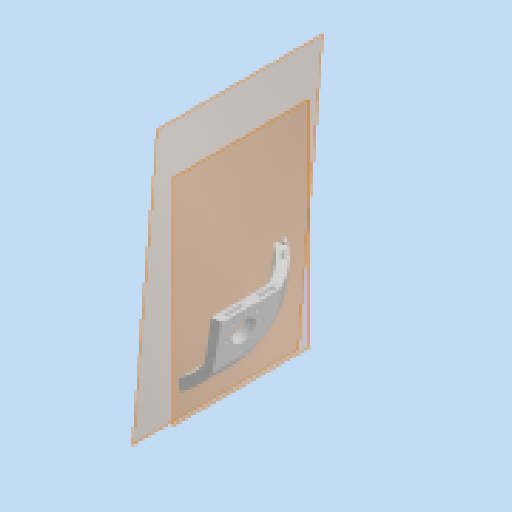
# Autodesk Inventor part: eggshellCorePrinted
Saved by Autodesk Inventor 2023 (Build 270158000, 158)
## iProperties
Created: 2026-03-19
Part Number: eggshellCorePrinted
Material: GFRC
Document SubType Name: Modeling
Designer: Nathann
Density: 1.7 g/cm^3
Appearance: Flat - Polished Gray
Mass: 25539 g
Surface Area: 11826.8 cm^2
Volume: 15023 cm^3
Author: Nathann
Autodesk Inventor part; units mm, degrees
ref_plane "XZ Plane" through (0, 0, 0) normal (0, 1, 0) x (-1, 0, 0)
ref_plane "XY Plane" through (0, 0, 0) normal (0, 0, 1) x (1, 0, 0)
sketch "Sketch1" plane through (0, 0, 0) normal (0, 0, 1) x (1, 0, 0)
  ellipse E0 centre (0, 0) end of major axis (0, 330) minor radius 450 (0, -330) -> (0, 330) ccw
  ellipse E1 centre (0, 0) end of major axis (420, 0) minor radius 300 (0, -300) -> (0, 300) ccw
  line L0 (0, 300) -> (0, 330)
  line L1 (0, -300) -> (0, -330)
  line L2 (420, 0) -> (450, 0)
  dimension "d0" = 420
  dimension "d1" = 450
  dimension "d2" = 300
  dimension "d3" = 330
  constraints: 6 end point, 2 coincident, 2 point on line, 1 horizontal, 10 other
extrude "Extrusion1" add sketch "Sketch1" along normal blind 80
sketch "Sketch2" plane through (0, 0, 80) normal (0, 0, 1) x (1, 0, 0)
  line L0 (0, 0) -> (451.5059, 0)
  ellipse E0 centre (0, 0) end of major axis (-450, 0) minor radius 330 (0, -330) -> (0, 330) ccw projected
  line L1 (0, 330) -> (0, 300) projected
  ellipse E1 centre (0, 0) end of major axis (-420, 0) minor radius 300 (0, -300) -> (0, 300) ccw projected
  line L2 (0, -300) -> (0, -330) projected
  point P0 (420, 0)
  point P1 (450, 0)
  constraints: 2 end point, 1 horizontal, 2 other
revolve "Revolution1" add sketch "Sketch2" angle 180 about axis through (0, 0, 80) along (1, 0, 0) contours E1 L1 E0 L0
sketch "Sketch3" plane through (0, 0, 0) normal (0, 0, -1) x (-1, 0, 0)
  ellipse E0 centre (0, 0) end of major axis (420, 0) minor radius 300 (0, 300) -> (0, -300) ccw projected
  line L0 (-410.6033, 63.104) -> (-375.8737, -133.8576)
  line L1 (-375.8737, -133.8576) -> (-428.5073, -143.1383)
  line L2 (-428.5073, -143.1383) -> (-456.291, 14.4309)
  line L3 (0, 300) -> (0, -300) projected
  ellipse E1 centre (0, 0) end of major axis (450, 0) minor radius 330 (0, 330) -> (0, -330) ccw projected
  line L4 (-456.291, 14.4309) -> (-439.6592, 70.3382)
  line L5 (-428.5073, -143.1383) -> (-336.4493, -219.1451)
  line L6 (-336.4493, -219.1451) -> (-375.8737, -133.8576)
  line L7 (-410.6033, 63.104) -> (-439.6592, 70.3382)
  line L8 (-393.2385, -35.3768) -> (260.9914, 90.2506)
  line L9 (260.9914, 90.2506) -> (260.9914, 44.7879)
  line L10 (260.9914, 44.7879) -> (0, 40.1342)
  dimension "d8" = 200
  dimension "d9" = 10
  dimension "d12" = 45.4627
  dimension "d13" = 160
  constraints: 20 end point, 2 perpendicular, 2 point on line, 1 midpoint, 1 vertical, 9 other
  measures "d8" distance of L0.start L0.end
  measures "d9" angle of L3 L0
  measures "d12" distance of L8.end L9.end
  measures "d13" distance of L1.end L2.end
extrude "Extrusion2" add sketch "Sketch3" against normal blind 190 contours L0 E0
ref_plane "Work Plane1" through (440.1475, 57.8945, 0) normal (-0.9848078, 0.1736482, 0) x (0, 0, 1)
sketch "Sketch5" plane through (440.1475, 57.8945, 0) normal (-0.9848078, 0.1736482, 0) x (0, 0, 1)
  line L0 (80, -458.4323) -> (80, -55.3041) projected
  circle A0 centre (80, -117.2866) radius 241.1725
  point P0 (0, -133.4458)
  constraints: 1 centre point, 1 point on line
extrude "Extrusion4" cut sketch "Sketch5" against normal blind 160
sketch "Sketch6" plane through (0, -330, 0) normal (-1, 0, 0) x (0, 0, 1)
  line L0 (0, 30) -> (0, 0) projected
  line L1 (0, 0) -> (80, 0) projected
  arc A0 (80, 0) -> (80, 660) centre (80, 330) ccw projected
  line L2 (0, 660) -> (80, 660) projected
  line L3 (0, 660) -> (0, 630) projected
  line L4 (0, 630) -> (80, 630) projected
  arc A1 (80, 30) -> (80, 630) centre (80, 330) ccw projected
  line L5 (0, 30) -> (80, 30) projected
  arc A2 (80, -50) -> (80, 710) centre (80, 330) ccw
  line L6 (80, -50) -> (-50, -50)
  line L7 (-50, -50) -> (-50, 80)
  line L8 (-50, 80) -> (80, 80)
  arc A3 (80, 80) -> (80, 580) centre (80, 330) ccw
  line L9 (80, 580) -> (-50, 580)
  line L10 (-50, 580) -> (-50, 710)
  line L11 (-50, 710) -> (80, 710)
  line L12 (0, 660) -> (0, 710)
  line L13 (0, 0) -> (0, -50)
  line L14 (80, 330) -> (410, 330)
  circle A4 centre (435, 330) radius 4.25
  circle A5 centre (426.0994, 408.9949) radius 4.25
  circle A6 centre (399.844, 484.0287) radius 4.25
  circle A7 centre (357.5502, 551.3389) radius 4.25
  circle A8 centre (301.3389, 607.5502) radius 4.25
  circle A9 centre (234.0288, 649.8439) radius 4.25
  circle A10 centre (158.995, 676.0994) radius 4.25
  circle A11 centre (80, 685) radius 4.25
  circle A12 centre (435, 330) radius 4.25
  circle A13 centre (426.0994, 251.0051) radius 4.25
  circle A14 centre (399.844, 175.9713) radius 4.25
  circle A15 centre (357.5502, 108.6611) radius 4.25
  circle A16 centre (301.3389, 52.4498) radius 4.25
  circle A17 centre (234.0288, 10.1561) radius 4.25
  circle A18 centre (158.995, -16.0994) radius 4.25
  circle A19 centre (80, -25) radius 4.25
  point P0 (0, 330)
  point P1 (460, 330)
  point P2 (80, -50)
  point P3 (460, 330)
  point P4 (439.25, 330)
  point P5 (430.75, 330)
  dimension "d19" = 50
  dimension "d22" = 8.5
  dimension "d25" = 90
  dimension "d27" = 25
  dimension "d28" = 0
  constraints: 18 centre point, 18 end point, 10 symmetric about line, 6 point on circle, 3 point on line, 1 perpendicular, 30 other
  measures "d19" distance between parallel lines of L1 L6
  measures "d22" diameter of A4
  measures "d27" distance of point (460, 330) A4.centre
  measures "d28" vertical distance of point (460, 330) A4.centre
extrude "Extrusion5" add sketch "Sketch6" against normal blind 10 contours L5 A1 L14 A0 L1 L0 | L1 A0 L2 L12 L11 A2 L6 L13 | A1 L4 L3 L2 A0 L14
ref_plane "Work Plane2" through (0, 0, 0) normal (0, 0, -1) x (-1, 0, 0)
mirror "Mirror1" about plane through (0, 0, 0) normal (0, 0, -1) of "Extrusion5", "Extrusion4", "Extrusion2", "Revolution1", "Extrusion1"
sketch "Sketch7" plane through (0, 0, 0) normal (0, 0, -1) x (-1, 0, 0)
  line L0 (-663.6694, -741.8919) -> (123.4449, -741.8919)
  line L1 (123.4449, -741.8919) -> (123.4449, 592.7802)
  line L2 (123.4449, 592.7802) -> (-663.6694, 592.7802)
  line L3 (-663.6694, 592.7802) -> (-663.6694, -741.8919)
  point P0 (0, 0)
  constraints: 8 end point, 2 parallel, 1 horizontal, 1 perpendicular
extrude "Extrusion6" cut sketch "Sketch7" against normal blind 1000
sketch "Sketch8" plane through (440.1475, 57.8945, 0) normal (0.9848078, -0.1736482, 0) x (0, 0, -1)
  line L0 (0, 6.7266) -> (80, 6.7266) projected
  line L1 (80, -205.7359) -> (0, -205.7359) projected
  circle A0 centre (80, -125.7359) radius 35
  line L2 (0, 6.7266) -> (0, -205.7359) projected
  circle A1 centre (80, -180.7359) radius 4.5
  circle A2 centre (118.8909, -164.6268) radius 4.5
  circle A3 centre (135, -125.7359) radius 4.5
  circle A4 centre (118.8909, -86.845) radius 4.5
  circle A5 centre (80, -70.7359) radius 4.5
  circle A6 centre (41.1091, -86.845) radius 4.5
  circle A7 centre (25, -125.7359) radius 4.5
  circle A8 centre (41.1091, -164.6268) radius 4.5
  point P0 (80.0002, -99.5046)
  dimension "d42" = 80
  dimension "d43" = 70
  dimension "d44" = 80
  dimension "d45" = 9
  dimension "d46" = 55
  dimension "d49" = 360
  constraints: 9 centre point, 1 vertical alignment, 17 other
  measures "d42" distance from line of L2 A0.centre
  measures "d43" diameter of A0
  measures "d44" distance from line of L1 A0.centre
  measures "d45" diameter of A1
  measures "d46" distance of A0.centre A1.centre
extrude "Extrusion7" cut sketch "Sketch8" against normal blind 50
ref_plane "Work Plane3" through (10, -2381.5933, 0) normal (0.9961947, -0.0871557, 0) x (0, 0, 1)
ref_plane "Work Plane4" through (300, 0, 0) normal (1, 0, 0) x (0, 1, 0)
sketch "Sketch10" plane through (300, 0, 0) normal (1, 0, 0) x (0, 1, 0)
  line L0 (-646.9693, -896.2791) -> (523.3446, -896.2791)
  line L1 (523.3446, -896.2791) -> (523.3446, 327.6055)
  line L2 (523.3446, 327.6055) -> (-646.9693, 327.6055)
  line L3 (-646.9693, 327.6055) -> (-646.9693, -896.2791)
  point P0 (0, 0)
  constraints: 8 end point, 2 parallel, 1 horizontal, 1 perpendicular
extrude "Extrusion9" cut sketch "Sketch10" against normal through all
sketch "Sketch11" plane through (300, 0, 0) normal (1, 0, 0) x (0, 1, 0)
  line L0 (384.5563, 0) -> (0.9675, 0)
  line L1 (0.9675, 0) -> (0.9675, -396.3946)
  line L2 (0.9675, -396.3946) -> (384.5563, -396.3946)
  line L3 (384.5563, -396.3946) -> (384.5563, 0)
  line L4 (245.9675, -80) -> (245.9675, 0) projected
  dimension "d58" = 245
  constraints: 8 end point, 2 parallel, 1 horizontal, 1 perpendicular
  measures "d58" distance between parallel lines of L1 L4
extrude "Extrusion10" cut sketch "Sketch11" along normal through all
sketch "Sketch12" plane through (399.647, 0.9675, 0) normal (0, 1, 0) x (1, 0, 0)
  line L0 (20.4628, 25) -> (10.4628, 25)
  line L1 (10.4628, 25) -> (10.4628, 75)
  line L2 (10.4628, 75) -> (20.4628, 75)
  line L3 (20.4628, 75) -> (20.4628, 25)
  line L4 (20.4628, 175) -> (10.4628, 175)
  line L5 (10.4628, 175) -> (10.4628, 125)
  line L6 (10.4628, 125) -> (20.4628, 125)
  line L7 (20.4628, 125) -> (20.4628, 175)
  line L8 (-61.515, 285.7558) -> (-26.1597, 250.4004)
  line L9 (-26.1597, 250.4004) -> (-33.2307, 243.3294)
  line L10 (-33.2307, 243.3294) -> (-68.5861, 278.6847)
  line L11 (-68.5861, 278.6847) -> (-61.515, 285.7558)
  line L12 (30.4628, 0) -> (0, 0) projected
  line L13 (30.4628, 177.0216) -> (30.4628, 0) projected
  line L14 (0, 0) -> (0, 172.2521) projected
  line L15 (-71.4051, 309.788) -> (19.6676, 218.7153)
  line L16 (-99.647, 0) -> (-23.7733, 0) projected
  line L17 (-36.7663, 275.1492) -> (-26.3833, 285.5322)
  point P0 (-399.647, 0)
  point P1 (0, 160)
  dimension "d59" = 10
  dimension "d60" = 10
  dimension "d61" = 50
  dimension "d62" = 50
  dimension "d63" = 10
  dimension "d64" = 50
  dimension "d65" = 25
  dimension "d66" = 50
  dimension "d67" = 10
  dimension "d68" = 10.4628
  dimension "d69" = 10
  dimension "d71" = 45
  dimension "d72" = 10
  dimension "d73" = 25
  constraints: 28 end point, 7 parallel, 4 perpendicular, 2 horizontal, 2 point on line, 3 other
  measures "d59" distance of L1.end L2.end
  measures "d60" distance of L4.start L4.end
  measures "d61" distance of L6.end L4.start
  measures "d62" distance of L2.end L0.start
  measures "d63" distance of L8.end L9.end
  measures "d64" distance of L8.start L8.end
  measures "d65" distance between parallel lines of L12 L0
  measures "d66" distance between parallel lines of L2 L6
  measures "d67" distance between parallel lines of L13 L3
  measures "d68" distance between parallel lines of L14 L1
  measures "d69" distance between parallel lines of L13 L7
  measures "d71" angle of L16 L15
  measures "d72" distance from line of L8 L17.start
  measures "d73" distance between parallel lines of L9 L17
extrude "Extrusion11" cut sketch "Sketch12" along normal blind 20 and the other way blind 20
sketch "Sketch13" plane through (300, 0, 0) normal (-1, 0, 0) x (0, 0, 1)
  line L0 (-25, -220.9675) -> (-75, -220.9675)
  line L1 (-75, -220.9675) -> (-75, -230.9675)
  line L2 (-75, -230.9675) -> (-25, -230.9675)
  line L3 (-25, -230.9675) -> (-25, -220.9675)
  line L4 (0, -245.9675) -> (-80, -245.9675) projected
  line L5 (0, -209.9563) -> (0, -245.9675) projected
  line L6 (-196.8684, -223.0235) -> (-238.1048, -188.422)
  line L7 (-247.6141, -160.8617) -> (-209.3119, -193.001)
  line L8 (-209.3119, -193.001) -> (-202.884, -185.3406)
  line L9 (-202.884, -185.3406) -> (-241.1863, -153.2012)
  line L10 (-241.1863, -153.2012) -> (-247.6141, -160.8617)
  line L11 (-247.6141, -160.8617) -> (-202.884, -185.3406) construction
  line L12 (-209.3119, -193.001) -> (-241.1863, -153.2012) construction
  line L13 (-238.1048, -188.422) -> (-256.0748, -209.8378)
  line L14 (-300.9656, -24.0325) -> (-310.9656, -24.0325)
  line L15 (-310.9656, -24.0325) -> (-310.9656, 25.9675)
  line L16 (-310.9656, 25.9675) -> (-300.9656, 25.9675)
  line L17 (-300.9656, 25.9675) -> (-300.9656, -24.0325)
  line L18 (-289.954, 0.9675) -> (-325.9656, 0.9675) projected
  point P0 (0, 0)
  point P1 (-225.2491, -173.1011)
  dimension "d78" = 10
  dimension "d79" = 50
  dimension "d80" = 15
  dimension "d81" = 25
  dimension "d90" = 50
  dimension "d91" = 50
  dimension "d92" = 10
  dimension "d93" = 25
  dimension "d94" = 15
  dimension "d95" = 10
  dimension "d96" = 50
  dimension "d97" = 25
  dimension "d98" = 15
  constraints: 32 end point, 6 parallel, 4 perpendicular, 2 horizontal, 2 midpoint, 3 other
  measures "d78" distance of L0.end L1.end
  measures "d79" distance of L1.end L2.end
  measures "d80" distance between parallel lines of L4 L2
  measures "d81" distance between parallel lines of L5 L3
  measures "d90" angle of L5 L6
  measures "d91" distance of L8.end L9.end
  measures "d92" distance of L9.end L7.start
  measures "d93" distance between parallel lines of L13 L10
  measures "d94" distance from line of L6.end L7
  measures "d95" distance of L14.start L14.end
  measures "d96" distance of L16.end L14.start
  measures "d97" distance between parallel lines of L18 L14
  measures "d98" distance from line of L15 L18.end
extrude "Extrusion12" cut sketch "Sketch13" against normal blind 20
fillet "Fillet1" radius 2 4 edges at (387.7603, -66.4451, 0) (417.2634, -71.8762, 0) (358.9109, -199.0604, 0) (342.1095, -174.0295, 0)
equation "\"d27\" = 0.5 * d19"
body "Solid1"
